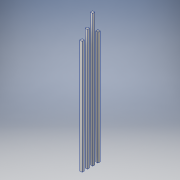
# Autodesk Inventor part: Legs
Saved by Autodesk Inventor 2019 (Build 230136000, 136)
## iProperties
Created: 2019-01-06
Part Number: Legs
Material: Aluminium 6061
Document SubType Name: Modeling
Designer: Jonas
Density: 2.7 g/cm^3
Appearance: Aluminium - flach
Author: Jonas
Autodesk Inventor part; units mm, degrees
ref_plane "YZ Plane" through (0, 0, 0) normal (1, 0, 0) x (0, 1, 0)
ref_plane "XZ Plane" through (0, 0, 0) normal (0, 1, 0) x (-1, 0, 0)
ref_plane "XY Plane" through (0, 0, 0) normal (0, 0, 1) x (1, 0, 0)
sketch "Skizze1" plane through (0, 0, 0) normal (1, 0, 0) x (0, 1, 0)
  line L0 (-11.2692, -2.1885) -> (-11.2692, -2.7885)
  line L1 (-11.2692, -2.7885) -> (18.7308, -2.7885)
  line L2 (18.7308, -2.7885) -> (18.7308, -2.1885)
  line L3 (18.7308, -2.1885) -> (-11.2692, -2.1885)
  line L4 (23.7308, -1.3885) -> (-11.2692, -1.3885)
  line L5 (-11.2692, -1.3885) -> (-11.2692, -0.7885)
  line L6 (-11.2692, -0.7885) -> (23.7308, -0.7885)
  line L7 (23.7308, -0.7885) -> (23.7308, -1.3885)
  line L8 (-11.2692, 0.0115) -> (-11.2692, 0.6115)
  line L9 (-11.2692, 0.6115) -> (20.7308, 0.6115)
  line L10 (20.7308, 0.6115) -> (20.7308, 0.0115)
  line L11 (20.7308, 0.0115) -> (-11.2692, 0.0115)
  line L12 (-11.2692, 0.8555) -> (-11.2692, 2.0115)
  line L13 (-11.2692, 2.0115) -> (18.7308, 2.0115)
  line L14 (18.7308, 2.0115) -> (18.7308, 1.4115)
  line L15 (18.7308, 1.4115) -> (-11.2692, 1.4115)
  point P0 (0, 0)
  dimension "d0" = 0.6
  dimension "d1" = 30
  dimension "d2" = 0.6
  dimension "d3" = 35
  dimension "d4" = 0.8
  dimension "d5" = 0.6
  dimension "d6" = 32
  dimension "d7" = 0.6
  dimension "d8" = 30
  dimension "d9" = 0.8
  dimension "d10" = 0.8
  constraints: 32 end point, 11 perpendicular, 3 vertical, 1 horizontal, 1 parallel, 1 point on line
  measures "d0" distance between parallel lines of L1 L3
  measures "d1" distance between parallel lines of L0 L2
  measures "d2" distance of L6.end L4.start
  measures "d3" distance between parallel lines of L5 L7
  measures "d4" distance between parallel lines of L4 L3
  measures "d5" distance of L9.end L10.end
  measures "d6" distance between parallel lines of L8 L10
  measures "d7" distance of L13.end L14.end
  measures "d8" distance between parallel lines of L12 L14
  measures "d9" distance between parallel lines of L11 L6
  measures "d10" distance between parallel lines of L15 L9
extrude "Extrusion1" add sketch "Skizze1" along normal blind 0.6
